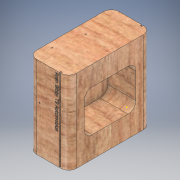
# Autodesk Inventor part: Passenger section
Saved by Autodesk Inventor 2017 (Build 210142000, 142)
## iProperties
Created: 2016-11-16
Part Number: Passenger section
Material: Wood (Birch)
Document SubType Name: Modeling
Designer: rbibb
Density: 0.55 g/cm^3
Appearance: Birch - Natural Polished
Author: rbibb
Autodesk Inventor part; units mm, degrees
ref_plane "YZ Plane" through (0, 0, 0) normal (1, 0, 0) x (0, 1, 0)
ref_plane "XZ Plane" through (0, 0, 0) normal (0, 1, 0) x (-1, 0, 0)
ref_plane "XY Plane" through (0, 0, 0) normal (0, 0, 1) x (1, 0, 0)
sketch "Sketch1" plane through (0, 0, 0) normal (1, 0, 0) x (0, 1, 0)
  line L0 (53.3666, 56.4874) -> (-27.1514, 56.4874)
  line L1 (-27.1514, 56.4874) -> (-27.1514, -24.0306)
  line L2 (-27.1514, -24.0306) -> (53.3666, -24.0306)
  line L3 (53.3666, -24.0306) -> (53.3666, 56.4874)
  point P0 (0, 0)
  dimension "d0" = 80.518
  dimension "d1" = 80.518
  constraints: 8 end point, 2 parallel, 1 horizontal, 1 perpendicular
  measures "d0" distance of L1.end L2.end
  measures "d1" distance of L2.end L0.start
extrude "Extrusion1" add sketch "Sketch1" along normal blind 38.862
sketch "Sketch4" plane through (38.862, 0, 0) normal (1, 0, 0) x (0, 0, -1)
  point P0 (0, 0)
sketch "Sketch5" plane through (38.862, 0, 0) normal (1, 0, 0) x (0, 0, -1)
  line L0 (-48.8674, -27.1514) -> (-56.4874, -27.1514) projected
  line L1 (-56.4874, -27.1514) -> (-56.4874, -6.3234)
  line L2 (-56.4874, 53.3666) -> (-56.4874, -27.1514) projected
  line L3 (-56.4874, -6.3234) -> (-41.2474, -6.3234)
  line L4 (-41.2474, -6.3234) -> (9.0446, -6.3234)
  line L5 (9.0446, -6.3234) -> (9.0446, 34.0626)
  line L6 (9.0446, 34.0626) -> (-41.2474, 34.0626)
  line L7 (-41.2474, 34.0626) -> (-41.2474, -6.3234)
  point P0 (0, 0)
  dimension "d9" = 20.828
  dimension "d10" = 15.24
  dimension "d11" = 50.292
  dimension "d12" = 40.386
  constraints: 12 end point, 2 parallel, 2 perpendicular, 1 horizontal, 1 point on line
  measures "d9" distance of L0.end L1.end
  measures "d10" distance of L1.end L3.end
  measures "d11" distance of L6.end L5.end
  measures "d12" distance of L5.end L4.end
extrude "Extrusion2" cut sketch "Sketch5" against normal blind 27.178
sketch "Sketch6" plane through (0, -27.1514, -16.4106) normal (0, -1, 0) x (1, 0, 0)
  point P0 (0, 16.4106)
sketch "Sketch7" plane through (0, -27.1514, -24.0306) normal (0, -1, 0) x (1, 0, 0)
  point P0 (0, 24.0306)
fillet "Fillet2" radius 7.62 4 edges at (38.862, 13.1076, -24.0306) (38.862, 13.1076, 56.4874) (0, 13.1076, -24.0306) (0, 13.1076, 56.4874)
sketch "Sketch8" plane through (0, -27.1514, -16.4106) normal (0, -1, 0) x (1, 0, 0)
  line L0 (7.62, 72.898) -> (31.242, 72.898) projected
  line L1 (7.62, 72.898) -> (7.62, 63.119)
  line L2 (7.62, 63.119) -> (30.48, 63.119)
  line L3 (30.48, 63.119) -> (30.48, 2.159)
  line L4 (30.48, 2.159) -> (7.62, 2.159)
  line L5 (7.62, 2.159) -> (7.62, 63.119)
  point P0 (0, 16.4106)
  dimension "d16" = 9.779
  dimension "d17" = 22.86
  dimension "d18" = 60.96
  constraints: 10 end point, 2 parallel, 1 horizontal, 1 perpendicular, 1 vertical
  measures "d16" distance of L0.start L1.end
  measures "d17" distance of L3.end L4.end
  measures "d18" distance of L2.end L3.end
extrude "Extrusion3" cut sketch "Sketch8" against normal blind 14.478
fillet "Fillet3" radius 7.62 4 edges at (7.62, -19.9124, 46.7084) (30.48, -19.9124, -14.2516) (30.48, -19.9124, 46.7084) (7.62, -19.9124, -14.2516)
fillet "Fillet4" radius 7.62 4 edges at (25.273, 34.0626, -9.0446) (25.273, 34.0626, 41.2474) (25.273, -6.3234, -9.0446) (25.273, -6.3234, 41.2474)
sketch "Sketch9" plane through (7.62, -27.1514, 56.4874) normal (0, 0, 1) x (1, 0, 0)
  line L0 (23.622, 80.518) -> (23.622, 0) projected
  line L1 (23.622, 80.518) -> (22.098, 80.518)
  line L2 (22.098, 80.518) -> (22.098, 0)
  line L3 (22.098, 0) -> (23.622, 0)
  line L4 (23.622, 0) -> (23.622, 80.518)
  point P0 (-7.62, 27.1514)
  dimension "d23" = 1.524
  constraints: 8 end point, 2 parallel, 1 horizontal, 1 perpendicular
  measures "d23" distance of L3.end L2.end
extrude "Extrusion4" cut sketch "Sketch9" against normal blind 1.524
sketch "Sketch10" plane through (7.62, -27.1514, 56.4874) normal (0, 0, 1) x (1, 0, 0)
  line L0 (18.2616, 76.5069) -> (18.2616, 77.0331)
  line L1 (18.2616, 77.0331) -> (19.4744, 77.9964)
  line L2 (19.4744, 77.9964) -> (19.4744, 78.4607)
  line L3 (19.4744, 78.4607) -> (18.2616, 78.4607)
  line L4 (18.2616, 78.4607) -> (18.2616, 78.8658)
  line L5 (18.2616, 78.8658) -> (21.3096, 78.8658)
  line L6 (21.3096, 78.8658) -> (21.3096, 78.0803)
  spline S0 degree 2 poles (21.3096, 78.0803) (21.3096, 77.8185) (21.2528, 77.4653) (21.149, 77.3048) knots 0 0 0 1 2 2 2
  spline S1 degree 2 poles (21.149, 77.3048) (21.0453, 77.1442) (20.7217, 76.959) (20.4821, 76.959) knots 0 0 0 1 2 2 2
  spline S2 degree 2 poles (20.4821, 76.959) (20.1487, 76.959) (19.6967, 77.2998) (19.588, 77.5913) knots 0 0 0 1 2 2 2
  line L7 (19.588, 77.5913) -> (18.2616, 76.5069)
  spline S3 degree 2 poles (20.45, 77.3813) (20.5834, 77.3813) (20.7884, 77.4752) (20.8551, 77.574) knots 0 0 0 1 2 2 2
  spline S4 degree 2 poles (20.8551, 77.574) (20.9119, 77.6604) (20.9588, 77.8902) (20.9588, 78.0581) knots 0 0 0 1 2 2 2
  line L8 (20.9588, 78.0581) -> (20.9588, 78.4607)
  line L9 (20.9588, 78.4607) -> (19.8128, 78.4607)
  line L10 (19.8128, 78.4607) -> (19.8128, 78.105)
  spline S5 degree 2 poles (19.8128, 78.105) (19.8128, 77.9297) (19.8745, 77.6506) (19.9708, 77.5542) knots 0 0 0 1 2 2 2
  spline S6 degree 2 poles (19.9708, 77.5542) (20.0548, 77.4653) (20.2919, 77.3813) (20.45, 77.3813) knots 0 0 0 1 2 2 2
  line L11 (20.5488, 74.4988) -> (17.4193, 75.7289)
  line L12 (17.4193, 75.7289) -> (17.4193, 76.1414)
  line L13 (17.4193, 76.1414) -> (18.3727, 75.7314)
  line L14 (18.3727, 75.7314) -> (20.5488, 76.5613)
  line L15 (20.5488, 76.5613) -> (20.5488, 76.1463)
  line L16 (20.5488, 76.1463) -> (18.8544, 75.5214)
  line L17 (18.8544, 75.5214) -> (20.5488, 74.899)
  line L18 (20.5488, 74.899) -> (20.5488, 74.4988)
  spline S7 degree 2 poles (18.5036, 72.9328) (18.4691, 72.9798) (18.3456, 73.1378) (18.3085, 73.2119) knots 0 0 0 1 2 2 2
  spline S8 degree 2 poles (18.3085, 73.2119) (18.2542, 73.3132) (18.1974, 73.5034) (18.1974, 73.6763) knots 0 0 0 1 2 2 2
  spline S9 degree 2 poles (18.1974, 73.6763) (18.1974, 73.8171) (18.3036, 74.0715) (18.3999, 74.1678) knots 0 0 0 1 2 2 2
  spline S10 degree 2 poles (18.3999, 74.1678) (18.4938, 74.2592) (18.7704, 74.3704) (18.9236, 74.3704) knots 0 0 0 1 2 2 2
  spline S11 degree 2 poles (18.9236, 74.3704) (19.1607, 74.3704) (19.4966, 74.1703) (19.5929, 73.953) knots 0 0 0 1 2 2 2
  spline S12 degree 2 poles (19.5929, 73.953) (19.6818, 73.7603) (19.7485, 73.2366) (19.7658, 72.9328) knots 0 0 0 1 2 2 2
  line L19 (19.7658, 72.9328) -> (19.8399, 72.9328)
  spline S13 degree 2 poles (19.8399, 72.9328) (19.9733, 72.9328) (20.1388, 73.0143) (20.1857, 73.0884) knots 0 0 0 1 2 2 2
  spline S14 degree 2 poles (20.1857, 73.0884) (20.2327, 73.1625) (20.2623, 73.375) (20.2623, 73.4886) knots 0 0 0 1 2 2 2
  spline S15 degree 2 poles (20.2623, 73.4886) (20.2623, 73.622) (20.1833, 73.9826) (20.1067, 74.1629) knots 0 0 0 1 2 2 2
  line L20 (20.1067, 74.1629) -> (20.1067, 74.1851)
  line L21 (20.1067, 74.1851) -> (20.4994, 74.1851)
  spline S16 degree 2 poles (20.4994, 74.1851) (20.5291, 74.0789) (20.6032, 73.6812) (20.6032, 73.4861) knots 0 0 0 1 2 2 2
  spline S17 degree 2 poles (20.6032, 73.4861) (20.6032, 73.249) (20.5291, 72.9254) (20.4327, 72.797) knots 0 0 0 1 2 2 2
  spline S18 degree 2 poles (20.4327, 72.797) (20.3389, 72.671) (20.04, 72.5475) (19.8251, 72.5475) knots 0 0 0 1 2 2 2
  line L22 (19.8251, 72.5475) -> (18.2616, 72.5475)
  line L23 (18.2616, 72.5475) -> (18.2616, 72.9328)
  line L24 (18.2616, 72.9328) -> (18.5036, 72.9328)
  line L25 (18.8247, 72.9328) -> (19.4595, 72.9328)
  spline S19 degree 2 poles (19.4595, 72.9328) (19.4472, 73.0712) (19.4052, 73.4886) (19.3657, 73.6195) knots 0 0 0 1 2 2 2
  spline S20 degree 2 poles (19.3657, 73.6195) (19.3188, 73.7726) (19.1236, 73.9727) (18.9507, 73.9727) knots 0 0 0 1 2 2 2
  spline S21 degree 2 poles (18.9507, 73.9727) (18.7531, 73.9727) (18.553, 73.7504) (18.553, 73.538) knots 0 0 0 1 2 2 2
  spline S22 degree 2 poles (18.553, 73.538) (18.553, 73.3577) (18.7087, 73.0613) (18.8247, 72.9328) knots 0 0 0 1 2 2 2
  line L26 (18.2616, 70.2109) -> (18.2616, 70.5962)
  line L27 (18.2616, 70.5962) -> (19.5658, 70.5962)
  spline S23 degree 2 poles (19.5658, 70.5962) (19.7238, 70.5962) (19.9955, 70.6258) (20.077, 70.6703) knots 0 0 0 1 2 2 2
  spline S24 degree 2 poles (20.077, 70.6703) (20.1635, 70.7172) (20.2475, 70.8852) (20.2475, 71.0285) knots 0 0 0 1 2 2 2
  spline S25 degree 2 poles (20.2475, 71.0285) (20.2475, 71.1717) (20.0943, 71.4755) (19.9708, 71.6213) knots 0 0 0 1 2 2 2
  line L28 (19.9708, 71.6213) -> (18.2616, 71.6213)
  line L29 (18.2616, 71.6213) -> (18.2616, 72.0066)
  line L30 (18.2616, 72.0066) -> (20.5488, 72.0066)
  line L31 (20.5488, 72.0066) -> (20.5488, 71.6213)
  line L32 (20.5488, 71.6213) -> (20.2944, 71.6213)
  spline S26 degree 2 poles (20.2944, 71.6213) (20.45, 71.4484) (20.613, 71.1149) (20.613, 70.9272) knots 0 0 0 1 2 2 2
  spline S27 degree 2 poles (20.613, 70.9272) (20.613, 70.5913) (20.1684, 70.2109) (19.7461, 70.2109) knots 0 0 0 1 2 2 2
  line L33 (19.7461, 70.2109) -> (18.2616, 70.2109)
  spline S28 degree 2 poles (19.1977, 66.2638) (18.9705, 66.2638) (18.6222, 66.4367) (18.5086, 66.58) knots 0 0 0 1 2 2 2
  spline S29 degree 2 poles (18.5086, 66.58) (18.3752, 66.7529) (18.2616, 67.1456) (18.2616, 67.4568) knots 0 0 0 1 2 2 2
  line L34 (18.2616, 67.4568) -> (18.2616, 68.3312)
  line L35 (18.2616, 68.3312) -> (21.3096, 68.3312)
  line L36 (21.3096, 68.3312) -> (21.3096, 67.5235)
  spline S30 degree 2 poles (21.3096, 67.5235) (21.3096, 67.1975) (21.2676, 66.8714) (21.1861, 66.7232) knots 0 0 0 1 2 2 2
  spline S31 degree 2 poles (21.1861, 66.7232) (21.0996, 66.5577) (20.8156, 66.4071) (20.6229, 66.4071) knots 0 0 0 1 2 2 2
  spline S32 degree 2 poles (20.6229, 66.4071) (20.408, 66.4071) (20.0672, 66.6343) (19.9708, 66.8344) knots 0 0 0 1 2 2 2
  line L37 (19.9708, 66.8344) -> (19.956, 66.8344)
  spline S33 degree 2 poles (19.956, 66.8344) (19.8819, 66.5627) (19.4892, 66.2638) (19.1977, 66.2638) knots 0 0 0 1 2 2 2
  spline S34 degree 2 poles (19.1804, 66.6862) (19.3533, 66.6862) (19.5756, 66.785) (19.6547, 66.9332) knots 0 0 0 1 2 2 2
  spline S35 degree 2 poles (19.6547, 66.9332) (19.7041, 67.0295) (19.7337, 67.2567) (19.7337, 67.4667) knots 0 0 0 1 2 2 2
  line L38 (19.7337, 67.4667) -> (19.7337, 67.9261)
  line L39 (19.7337, 67.9261) -> (18.6074, 67.9261)
  line L40 (18.6074, 67.9261) -> (18.6074, 67.5976)
  spline S36 degree 2 poles (18.6074, 67.5976) (18.6074, 67.3308) (18.6568, 67.0246) (18.7358, 66.906) knots 0 0 0 1 2 2 2
  spline S37 degree 2 poles (18.7358, 66.906) (18.8173, 66.7924) (19.0199, 66.6862) (19.1804, 66.6862) knots 0 0 0 1 2 2 2
  spline S38 degree 2 poles (20.5661, 66.8294) (20.6748, 66.8294) (20.8378, 66.9035) (20.8847, 66.985) knots 0 0 0 1 2 2 2
  spline S39 degree 2 poles (20.8847, 66.985) (20.9391, 67.0838) (20.9638, 67.3234) (20.9638, 67.5383) knots 0 0 0 1 2 2 2
  line L41 (20.9638, 67.5383) -> (20.9638, 67.9261)
  line L42 (20.9638, 67.9261) -> (20.0721, 67.9261)
  line L43 (20.0721, 67.9261) -> (20.0721, 67.4667)
  spline S40 degree 2 poles (20.0721, 67.4667) (20.0721, 67.2765) (20.1116, 67.0962) (20.1734, 66.9999) knots 0 0 0 1 2 2 2
  spline S41 degree 2 poles (20.1734, 66.9999) (20.2327, 66.906) (20.4229, 66.8294) (20.5661, 66.8294) knots 0 0 0 1 2 2 2
  line L44 (18.2616, 65.4981) -> (18.2616, 65.8834)
  line L45 (18.2616, 65.8834) -> (20.5488, 65.8834)
  line L46 (20.5488, 65.8834) -> (20.5488, 65.4981)
  line L47 (20.5488, 65.4981) -> (18.2616, 65.4981)
  line L48 (20.9292, 65.4709) -> (20.9292, 65.9081)
  line L49 (20.9292, 65.9081) -> (21.3293, 65.9081)
  line L50 (21.3293, 65.9081) -> (21.3293, 65.4709)
  line L51 (21.3293, 65.4709) -> (20.9292, 65.4709)
  spline S42 degree 2 poles (19.4423, 63.0157) (18.8816, 63.0157) (18.1974, 63.5591) (18.1974, 63.9691) knots 0 0 0 1 2 2 2
  spline S43 degree 2 poles (18.1974, 63.9691) (18.1974, 64.1544) (18.2888, 64.4187) (18.3678, 64.5471) knots 0 0 0 1 2 2 2
  line L52 (18.3678, 64.5471) -> (18.2616, 64.5718)
  line L53 (18.2616, 64.5718) -> (18.2616, 64.9325)
  line L54 (18.2616, 64.9325) -> (21.4454, 64.9325)
  line L55 (21.4454, 64.9325) -> (21.4454, 64.5471)
  line L56 (21.4454, 64.5471) -> (20.3092, 64.5471)
  spline S44 degree 2 poles (20.3092, 64.5471) (20.4401, 64.4014) (20.613, 64.063) (20.613, 63.8481) knots 0 0 0 1 2 2 2
  spline S45 degree 2 poles (20.613, 63.8481) (20.613, 63.4603) (19.9931, 63.0157) (19.4423, 63.0157) knots 0 0 0 1 2 2 2
  spline S46 degree 2 poles (19.4126, 63.4134) (19.8226, 63.4134) (20.2475, 63.6629) (20.2475, 63.9395) knots 0 0 0 1 2 2 2
  spline S47 degree 2 poles (20.2475, 63.9395) (20.2475, 64.0951) (20.0993, 64.4162) (19.9857, 64.5471) knots 0 0 0 1 2 2 2
  line L57 (19.9857, 64.5471) -> (18.6741, 64.5471)
  spline S48 degree 2 poles (18.6741, 64.5471) (18.6024, 64.4014) (18.5432, 64.1766) (18.5432, 64.0432) knots 0 0 0 1 2 2 2
  spline S49 degree 2 poles (18.5432, 64.0432) (18.5432, 63.7493) (18.9606, 63.4134) (19.4126, 63.4134) knots 0 0 0 1 2 2 2
  spline S50 degree 2 poles (19.4423, 60.6988) (18.8816, 60.6988) (18.1974, 61.2422) (18.1974, 61.6523) knots 0 0 0 1 2 2 2
  spline S51 degree 2 poles (18.1974, 61.6523) (18.1974, 61.8375) (18.2888, 62.1018) (18.3678, 62.2303) knots 0 0 0 1 2 2 2
  line L58 (18.3678, 62.2303) -> (18.2616, 62.255)
  line L59 (18.2616, 62.255) -> (18.2616, 62.6156)
  line L60 (18.2616, 62.6156) -> (21.4454, 62.6156)
  line L61 (21.4454, 62.6156) -> (21.4454, 62.2303)
  line L62 (21.4454, 62.2303) -> (20.3092, 62.2303)
  spline S52 degree 2 poles (20.3092, 62.2303) (20.4401, 62.0845) (20.613, 61.7461) (20.613, 61.5312) knots 0 0 0 1 2 2 2
  spline S53 degree 2 poles (20.613, 61.5312) (20.613, 61.1434) (19.9931, 60.6988) (19.4423, 60.6988) knots 0 0 0 1 2 2 2
  spline S54 degree 2 poles (19.4126, 61.0965) (19.8226, 61.0965) (20.2475, 61.346) (20.2475, 61.6226) knots 0 0 0 1 2 2 2
  spline S55 degree 2 poles (20.2475, 61.6226) (20.2475, 61.7782) (20.0993, 62.0993) (19.9857, 62.2303) knots 0 0 0 1 2 2 2
  line L63 (19.9857, 62.2303) -> (18.6741, 62.2303)
  spline S56 degree 2 poles (18.6741, 62.2303) (18.6024, 62.0845) (18.5432, 61.8598) (18.5432, 61.7264) knots 0 0 0 1 2 2 2
  spline S57 degree 2 poles (18.5432, 61.7264) (18.5432, 61.4324) (18.9606, 61.0965) (19.4126, 61.0965) knots 0 0 0 1 2 2 2
  line L64 (20.5488, 58.503) -> (17.4193, 59.7331)
  line L65 (17.4193, 59.7331) -> (17.4193, 60.1456)
  line L66 (17.4193, 60.1456) -> (18.3727, 59.7355)
  line L67 (18.3727, 59.7355) -> (20.5488, 60.5655)
  line L68 (20.5488, 60.5655) -> (20.5488, 60.1505)
  line L69 (20.5488, 60.1505) -> (18.8544, 59.5256)
  line L70 (18.8544, 59.5256) -> (20.5488, 58.9031)
  line L71 (20.5488, 58.9031) -> (20.5488, 58.503)
  line L72 (18.2616, 56.1614) -> (20.949, 56.1614)
  line L73 (20.949, 56.1614) -> (20.949, 57.184)
  line L74 (20.949, 57.184) -> (21.3096, 57.184)
  line L75 (21.3096, 57.184) -> (21.3096, 54.7338)
  line L76 (21.3096, 54.7338) -> (20.949, 54.7338)
  line L77 (20.949, 54.7338) -> (20.949, 55.7563)
  line L78 (20.949, 55.7563) -> (18.2616, 55.7563)
  line L79 (18.2616, 55.7563) -> (18.2616, 56.1614)
  spline S58 degree 2 poles (20.3191, 54.5954) (20.5538, 54.5954) (20.944, 54.4423) (21.0848, 54.3089) knots 0 0 0 1 2 2 2
  spline S59 degree 2 poles (21.0848, 54.3089) (21.2207, 54.1829) (21.3713, 53.8149) (21.3713, 53.6272) knots 0 0 0 1 2 2 2
  spline S60 degree 2 poles (21.3713, 53.6272) (21.3713, 53.4172) (21.2305, 53.0764) (21.0972, 52.9504) knots 0 0 0 1 2 2 2
  spline S61 degree 2 poles (21.0972, 52.9504) (20.9292, 52.7923) (20.3858, 52.6194) (19.9684, 52.6194) knots 0 0 0 1 2 2 2
  spline S62 degree 2 poles (19.9684, 52.6194) (19.5905, 52.6194) (18.9137, 52.7899) (18.6889, 52.9553) knots 0 0 0 1 2 2 2
  spline S63 degree 2 poles (18.6889, 52.9553) (18.4518, 53.1307) (18.2023, 53.6247) (18.2023, 53.9853) knots 0 0 0 1 2 2 2
  spline S64 degree 2 poles (18.2023, 53.9853) (18.2023, 54.0669) (18.2196, 54.2521) (18.2443, 54.3311) knots 0 0 0 1 2 2 2
  line L80 (18.2443, 54.3311) -> (18.637, 54.3311)
  line L81 (18.637, 54.3311) -> (18.637, 54.3114)
  spline S65 degree 2 poles (18.637, 54.3114) (18.6074, 54.2595) (18.5555, 54.0422) (18.5555, 53.931) knots 0 0 0 1 2 2 2
  spline S66 degree 2 poles (18.5555, 53.931) (18.5555, 53.5309) (19.0841, 53.0739) (19.5732, 53.0418) knots 0 0 0 1 2 2 2
  spline S67 degree 2 poles (19.5732, 53.0418) (19.462, 53.2048) (19.3607, 53.5012) (19.3607, 53.6766) knots 0 0 0 1 2 2 2
  spline S68 degree 2 poles (19.3607, 53.6766) (19.3607, 53.8445) (19.4348, 54.1237) (19.5411, 54.2645) knots 0 0 0 1 2 2 2
  spline S69 degree 2 poles (19.5411, 54.2645) (19.667, 54.4275) (20.0499, 54.5954) (20.3191, 54.5954) knots 0 0 0 1 2 2 2
  spline S70 degree 2 poles (20.0598, 53.0319) (20.3685, 53.0319) (20.7588, 53.1455) (20.865, 53.2468) knots 0 0 0 1 2 2 2
  spline S71 degree 2 poles (20.865, 53.2468) (20.9638, 53.3357) (21.0379, 53.521) (21.0379, 53.6297) knots 0 0 0 1 2 2 2
  spline S72 degree 2 poles (21.0379, 53.6297) (21.0379, 53.8816) (20.6773, 54.1805) (20.3364, 54.1805) knots 0 0 0 1 2 2 2
  spline S73 degree 2 poles (20.3364, 54.1805) (20.1437, 54.1805) (19.8943, 54.0817) (19.8053, 53.973) knots 0 0 0 1 2 2 2
  spline S74 degree 2 poles (19.8053, 53.973) (19.7411, 53.8939) (19.6991, 53.6988) (19.6991, 53.5852) knots 0 0 0 1 2 2 2
  spline S75 degree 2 poles (19.6991, 53.5852) (19.6991, 53.4543) (19.7905, 53.1529) (19.8671, 53.0393) knots 0 0 0 1 2 2 2
  spline S76 degree 2 poles (19.8671, 53.0393) (19.8967, 53.0369) (19.998, 53.0319) (20.0598, 53.0319) knots 0 0 0 1 2 2 2
  line L82 (18.2616, 51.1572) -> (21.3096, 50.1296)
  line L83 (21.3096, 50.1296) -> (21.3096, 49.6307)
  line L84 (21.3096, 49.6307) -> (18.2616, 48.6032)
  line L85 (18.2616, 48.6032) -> (18.2616, 49.0305)
  line L86 (18.2616, 49.0305) -> (19.1137, 49.3071)
  line L87 (19.1137, 49.3071) -> (19.1137, 50.4705)
  line L88 (19.1137, 50.4705) -> (18.2616, 50.7471)
  line L89 (18.2616, 50.7471) -> (18.2616, 51.1572)
  line L90 (19.4595, 49.4183) -> (20.8946, 49.8901)
  line L91 (20.8946, 49.8901) -> (19.4595, 50.3594)
  line L92 (19.4595, 50.3594) -> (19.4595, 49.4183)
  line L93 (18.2616, 46.5654) -> (18.2616, 46.9507)
  line L94 (18.2616, 46.9507) -> (18.5135, 46.9507)
  spline S77 degree 2 poles (18.5135, 46.9507) (18.3579, 47.1286) (18.1974, 47.4472) (18.1974, 47.6448) knots 0 0 0 1 2 2 2
  spline S78 degree 2 poles (18.1974, 47.6448) (18.1974, 47.793) (18.2962, 48.0573) (18.4024, 48.1536) knots 0 0 0 1 2 2 2
  spline S79 degree 2 poles (18.4024, 48.1536) (18.5086, 48.2524) (18.8322, 48.3611) (19.0643, 48.3611) knots 0 0 0 1 2 2 2
  line L95 (19.0643, 48.3611) -> (20.5488, 48.3611)
  line L96 (20.5488, 48.3611) -> (20.5488, 47.9758)
  line L97 (20.5488, 47.9758) -> (19.2447, 47.9758)
  spline S80 degree 2 poles (19.2447, 47.9758) (19.0619, 47.9758) (18.8223, 47.9486) (18.7334, 47.9017) knots 0 0 0 1 2 2 2
  spline S81 degree 2 poles (18.7334, 47.9017) (18.6444, 47.8548) (18.5629, 47.6942) (18.5629, 47.5435) knots 0 0 0 1 2 2 2
  spline S82 degree 2 poles (18.5629, 47.5435) (18.5629, 47.4027) (18.7235, 47.0841) (18.8396, 46.9507) knots 0 0 0 1 2 2 2
  line L98 (18.8396, 46.9507) -> (20.5488, 46.9507)
  line L99 (20.5488, 46.9507) -> (20.5488, 46.5654)
  line L100 (20.5488, 46.5654) -> (18.2616, 46.5654)
  spline S83 degree 2 poles (18.2171, 45.3156) (18.2171, 45.6293) (18.5753, 45.9825) (18.9631, 45.9825) knots 0 0 0 1 2 2 2
  line L101 (18.9631, 45.9825) -> (20.2302, 45.9825)
  line L102 (20.2302, 45.9825) -> (20.2302, 46.2418)
  line L103 (20.2302, 46.2418) -> (20.5488, 46.2418)
  line L104 (20.5488, 46.2418) -> (20.5488, 45.9825)
  line L105 (20.5488, 45.9825) -> (21.2058, 45.9825)
  line L106 (21.2058, 45.9825) -> (21.2058, 45.5972)
  line L107 (21.2058, 45.5972) -> (20.5488, 45.5972)
  line L108 (20.5488, 45.5972) -> (20.5488, 44.8883)
  line L109 (20.5488, 44.8883) -> (20.2302, 44.8883)
  line L110 (20.2302, 44.8883) -> (20.2302, 45.5972)
  line L111 (20.2302, 45.5972) -> (19.1409, 45.5972)
  spline S84 degree 2 poles (19.1409, 45.5972) (18.968, 45.5972) (18.7778, 45.5848) (18.6963, 45.5428) knots 0 0 0 1 2 2 2
  spline S85 degree 2 poles (18.6963, 45.5428) (18.6247, 45.5082) (18.553, 45.3526) (18.553, 45.2193) knots 0 0 0 1 2 2 2
  spline S86 degree 2 poles (18.553, 45.2193) (18.553, 45.1254) (18.6099, 44.95) (18.6271, 44.9105) knots 0 0 0 1 2 2 2
  line L112 (18.6271, 44.9105) -> (18.6271, 44.8883)
  line L113 (18.6271, 44.8883) -> (18.2813, 44.8883)
  spline S87 degree 2 poles (18.2813, 44.8883) (18.2517, 44.997) (18.2171, 45.2193) (18.2171, 45.3156) knots 0 0 0 1 2 2 2
  spline S88 degree 2 poles (19.4052, 42.7245) (18.8272, 42.7245) (18.1974, 43.2803) (18.1974, 43.7447) knots 0 0 0 1 2 2 2
  spline S89 degree 2 poles (18.1974, 43.7447) (18.1974, 44.2214) (18.847, 44.7672) (19.4052, 44.7672) knots 0 0 0 1 2 2 2
  spline S90 degree 2 poles (19.4052, 44.7672) (19.9782, 44.7672) (20.613, 44.2041) (20.613, 43.7447) knots 0 0 0 1 2 2 2
  spline S91 degree 2 poles (20.613, 43.7447) (20.613, 43.2803) (19.9807, 42.7245) (19.4052, 42.7245) knots 0 0 0 1 2 2 2
  spline S92 degree 2 poles (19.4052, 43.1222) (19.8498, 43.1222) (20.2821, 43.4458) (20.2821, 43.7447) knots 0 0 0 1 2 2 2
  spline S93 degree 2 poles (20.2821, 43.7447) (20.2821, 44.0435) (19.8498, 44.3696) (19.4052, 44.3696) knots 0 0 0 1 2 2 2
  spline S94 degree 2 poles (19.4052, 44.3696) (18.973, 44.3696) (18.5283, 44.0435) (18.5283, 43.7447) knots 0 0 0 1 2 2 2
  spline S95 degree 2 poles (18.5283, 43.7447) (18.5283, 43.4483) (18.9655, 43.1222) (19.4052, 43.1222) knots 0 0 0 1 2 2 2
  line L114 (18.2616, 39.7358) -> (19.5855, 39.7358)
  spline S96 degree 2 poles (19.5855, 39.7358) (19.7436, 39.7358) (20.0128, 39.7605) (20.0869, 39.8) knots 0 0 0 1 2 2 2
  spline S97 degree 2 poles (20.0869, 39.8) (20.1684, 39.8396) (20.2475, 39.9902) (20.2475, 40.1211) knots 0 0 0 1 2 2 2
  spline S98 degree 2 poles (20.2475, 40.1211) (20.2475, 40.2397) (20.1017, 40.5114) (19.9634, 40.6547) knots 0 0 0 1 2 2 2
  spline S99 degree 2 poles (19.9634, 40.6547) (19.9288, 40.6522) (19.8325, 40.6473) (19.7683, 40.6473) knots 0 0 0 1 2 2 2
  line L115 (19.7683, 40.6473) -> (18.2616, 40.6473)
  line L116 (18.2616, 40.6473) -> (18.2616, 41.0326)
  line L117 (18.2616, 41.0326) -> (19.5855, 41.0326)
  spline S100 degree 2 poles (19.5855, 41.0326) (19.7436, 41.0326) (20.0128, 41.0573) (20.0869, 41.0968) knots 0 0 0 1 2 2 2
  spline S101 degree 2 poles (20.0869, 41.0968) (20.1684, 41.1363) (20.2475, 41.287) (20.2475, 41.4179) knots 0 0 0 1 2 2 2
  spline S102 degree 2 poles (20.2475, 41.4179) (20.2475, 41.5414) (20.0919, 41.8156) (19.9708, 41.944) knots 0 0 0 1 2 2 2
  line L118 (19.9708, 41.944) -> (18.2616, 41.944)
  line L119 (18.2616, 41.944) -> (18.2616, 42.3293)
  line L120 (18.2616, 42.3293) -> (20.5488, 42.3293)
  line L121 (20.5488, 42.3293) -> (20.5488, 41.944)
  line L122 (20.5488, 41.944) -> (20.2969, 41.944)
  spline S103 degree 2 poles (20.2969, 41.944) (20.4476, 41.7933) (20.613, 41.4969) (20.613, 41.3191) knots 0 0 0 1 2 2 2
  spline S104 degree 2 poles (20.613, 41.3191) (20.613, 41.1166) (20.4278, 40.8029) (20.2178, 40.7214) knots 0 0 0 1 2 2 2
  spline S105 degree 2 poles (20.2178, 40.7214) (20.413, 40.546) (20.613, 40.215) (20.613, 40.0223) knots 0 0 0 1 2 2 2
  spline S106 degree 2 poles (20.613, 40.0223) (20.613, 39.8741) (20.5217, 39.6321) (20.4179, 39.5432) knots 0 0 0 1 2 2 2
  spline S107 degree 2 poles (20.4179, 39.5432) (20.3142, 39.4518) (20.0029, 39.3505) (19.7683, 39.3505) knots 0 0 0 1 2 2 2
  line L123 (19.7683, 39.3505) -> (18.2616, 39.3505)
  line L124 (18.2616, 39.3505) -> (18.2616, 39.7358)
  spline S108 degree 2 poles (19.4052, 36.9299) (18.8272, 36.9299) (18.1974, 37.4856) (18.1974, 37.95) knots 0 0 0 1 2 2 2
  spline S109 degree 2 poles (18.1974, 37.95) (18.1974, 38.4267) (18.847, 38.9726) (19.4052, 38.9726) knots 0 0 0 1 2 2 2
  spline S110 degree 2 poles (19.4052, 38.9726) (19.9782, 38.9726) (20.613, 38.4094) (20.613, 37.95) knots 0 0 0 1 2 2 2
  spline S111 degree 2 poles (20.613, 37.95) (20.613, 37.4856) (19.9807, 36.9299) (19.4052, 36.9299) knots 0 0 0 1 2 2 2
  spline S112 degree 2 poles (19.4052, 37.3276) (19.8498, 37.3276) (20.2821, 37.6511) (20.2821, 37.95) knots 0 0 0 1 2 2 2
  spline S113 degree 2 poles (20.2821, 37.95) (20.2821, 38.2489) (19.8498, 38.5749) (19.4052, 38.5749) knots 0 0 0 1 2 2 2
  spline S114 degree 2 poles (19.4052, 38.5749) (18.973, 38.5749) (18.5283, 38.2489) (18.5283, 37.95) knots 0 0 0 1 2 2 2
  spline S115 degree 2 poles (18.5283, 37.95) (18.5283, 37.6536) (18.9655, 37.3276) (19.4052, 37.3276) knots 0 0 0 1 2 2 2
  spline S116 degree 2 poles (19.4423, 34.6179) (18.8816, 34.6179) (18.1974, 35.1613) (18.1974, 35.5714) knots 0 0 0 1 2 2 2
  spline S117 degree 2 poles (18.1974, 35.5714) (18.1974, 35.7566) (18.2888, 36.0209) (18.3678, 36.1494) knots 0 0 0 1 2 2 2
  line L125 (18.3678, 36.1494) -> (18.2616, 36.1741)
  line L126 (18.2616, 36.1741) -> (18.2616, 36.5347)
  line L127 (18.2616, 36.5347) -> (21.4454, 36.5347)
  line L128 (21.4454, 36.5347) -> (21.4454, 36.1494)
  line L129 (21.4454, 36.1494) -> (20.3092, 36.1494)
  spline S118 degree 2 poles (20.3092, 36.1494) (20.4401, 36.0036) (20.613, 35.6652) (20.613, 35.4503) knots 0 0 0 1 2 2 2
  spline S119 degree 2 poles (20.613, 35.4503) (20.613, 35.0625) (19.9931, 34.6179) (19.4423, 34.6179) knots 0 0 0 1 2 2 2
  spline S120 degree 2 poles (19.4126, 35.0156) (19.8226, 35.0156) (20.2475, 35.2651) (20.2475, 35.5417) knots 0 0 0 1 2 2 2
  spline S121 degree 2 poles (20.2475, 35.5417) (20.2475, 35.6973) (20.0993, 36.0184) (19.9857, 36.1494) knots 0 0 0 1 2 2 2
  line L130 (19.9857, 36.1494) -> (18.6741, 36.1494)
  spline S122 degree 2 poles (18.6741, 36.1494) (18.6024, 36.0036) (18.5432, 35.7789) (18.5432, 35.6455) knots 0 0 0 1 2 2 2
  spline S123 degree 2 poles (18.5432, 35.6455) (18.5432, 35.3515) (18.9606, 35.0156) (19.4126, 35.0156) knots 0 0 0 1 2 2 2
  line L131 (18.2616, 33.8251) -> (18.2616, 34.2104)
  line L132 (18.2616, 34.2104) -> (21.4454, 34.2104)
  line L133 (21.4454, 34.2104) -> (21.4454, 33.8251)
  line L134 (21.4454, 33.8251) -> (18.2616, 33.8251)
  spline S124 degree 2 poles (19.4052, 31.3798) (18.8272, 31.3798) (18.1974, 31.9355) (18.1974, 32.3999) knots 0 0 0 1 2 2 2
  spline S125 degree 2 poles (18.1974, 32.3999) (18.1974, 32.8766) (18.847, 33.4225) (19.4052, 33.4225) knots 0 0 0 1 2 2 2
  spline S126 degree 2 poles (19.4052, 33.4225) (19.9782, 33.4225) (20.613, 32.8593) (20.613, 32.3999) knots 0 0 0 1 2 2 2
  spline S127 degree 2 poles (20.613, 32.3999) (20.613, 31.9355) (19.9807, 31.3798) (19.4052, 31.3798) knots 0 0 0 1 2 2 2
  spline S128 degree 2 poles (19.4052, 31.7774) (19.8498, 31.7774) (20.2821, 32.101) (20.2821, 32.3999) knots 0 0 0 1 2 2 2
  spline S129 degree 2 poles (20.2821, 32.3999) (20.2821, 32.6987) (19.8498, 33.0248) (19.4052, 33.0248) knots 0 0 0 1 2 2 2
  spline S130 degree 2 poles (19.4052, 33.0248) (18.973, 33.0248) (18.5283, 32.6987) (18.5283, 32.3999) knots 0 0 0 1 2 2 2
  spline S131 degree 2 poles (18.5283, 32.3999) (18.5283, 32.1035) (18.9655, 31.7774) (19.4052, 31.7774) knots 0 0 0 1 2 2 2
  line L135 (18.2616, 29.2086) -> (18.2616, 29.6804)
  line L136 (18.2616, 29.6804) -> (19.1212, 30.2361)
  line L137 (19.1212, 30.2361) -> (18.2616, 30.8067)
  line L138 (18.2616, 30.8067) -> (18.2616, 31.2439)
  line L139 (18.2616, 31.2439) -> (19.3953, 30.451)
  line L140 (19.3953, 30.451) -> (20.5488, 31.2365)
  line L141 (20.5488, 31.2365) -> (20.5488, 30.7647)
  line L142 (20.5488, 30.7647) -> (19.6967, 30.2114)
  line L143 (19.6967, 30.2114) -> (20.5488, 29.6458)
  line L144 (20.5488, 29.6458) -> (20.5488, 29.2086)
  line L145 (20.5488, 29.2086) -> (19.42, 29.9965)
  line L146 (19.42, 29.9965) -> (18.2616, 29.2086)
  point P0 (-7.62, 27.1514)
  point P1 (21.4454, 79.1746)
  constraints: 1 other
emboss "Emboss1" sketch "Sketch10" operation cut depth 1.27 direction (0, 0, -1)
sketch "Sketch11" plane through (31.242, 53.3666, -24.0306) normal (0, 0, -1) x (-1, 0, 0)
  line L0 (0, -80.518) -> (-7.62, -80.518) projected
  line L1 (23.622, 0) -> (1.524, 0) projected
  line L2 (0, -80.518) -> (1.524, -80.518)
  line L3 (1.524, -80.518) -> (1.524, 0)
  line L4 (1.524, 0) -> (0, 0)
  line L5 (0, 0) -> (0, -80.518)
  point P0 (31.242, -53.3666)
  constraints: 8 end point, 2 parallel, 1 horizontal, 1 perpendicular
extrude "Extrusion5" cut sketch "Sketch11" against normal blind 1.524
body "Solid1"
